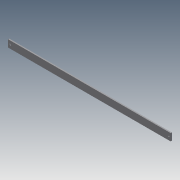
# Autodesk Inventor part: large
Saved by Autodesk Inventor 2011 (Build 150239000, 239)
## iProperties
Created: 2011-12-18
Part Number: large
Document SubType Name: Modeling
Designer: Matthew
Density: 1 g/cm^3
Author: Matthew
Autodesk Inventor part; units mm, degrees
ref_plane "YZ Plane" through (0, 0, 0) normal (1, 0, 0) x (0, 1, 0)
ref_plane "XZ Plane" through (0, 0, 0) normal (0, 1, 0) x (-1, 0, 0)
ref_plane "XY Plane" through (0, 0, 0) normal (0, 0, 1) x (1, 0, 0)
sketch "Sketch1" plane through (0, 0, 0) normal (0, 0, 1) x (1, 0, 0)
  line L0 (-31.9376, 1.7652) -> (399.8624, 1.7652)
  line L1 (399.8624, 1.7652) -> (399.8624, -10.9348)
  line L2 (399.8624, -10.9348) -> (-31.9376, -10.9348)
  line L3 (-31.9376, -10.9348) -> (-31.9376, 1.7652)
  line L4 (183.9624, -4.5848) -> (-26.4766, -4.5848)
  line L5 (-26.4766, -4.5848) -> (394.4014, -4.5848)
  circle A0 centre (-26.4766, -4.5848) radius 1.9812
  circle A1 centre (394.4014, -4.5848) radius 1.9812
  point P0 (0, 0)
  dimension "d0" = 431.8
  dimension "d1" = 12.7
  dimension "d2" = 210.439
  dimension "d3" = 420.878
  dimension "d4" = 3.9624
  dimension "d5" = 3.9624
  constraints: 12 end point, 3 parallel, 2 centre point, 2 coincident, 2 perpendicular, 1 horizontal
  measures "d0" distance of L1.end L2.end
  measures "d1" distance of L0.end L1.end
  measures "d2" distance of L4.start L4.end
  measures "d3" distance of L4.end L5.end
  measures "d4" diameter of A0
  measures "d5" diameter of A1
extrude "Extrusion1" add sketch "Sketch1" along normal blind 3.175
sketch "Sketch2" plane through (-31.9376, 1.7652, 0) normal (0, 1, 0) x (1, 0, 0)
  line L0 (0, -3.175) -> (431.8, -3.175) projected
  line L1 (431.8, 0) -> (431.8, -3.175) projected
  line L2 (0, 0) -> (431.8, 0) projected
  line L3 (0, 0) -> (0, -3.175) projected
  point P0 (31.9376, 0)
extrude "Extrusion2" add sketch "Sketch2" along normal blind 3.175
sketch "Sketch3" plane through (-31.9376, -10.9348, 0) normal (0, -1, 0) x (1, 0, 0)
  line L0 (431.8, 3.175) -> (0, 3.175) projected
  line L1 (0, 0) -> (0, 3.175) projected
  line L2 (431.8, 0) -> (0, 0) projected
  line L3 (431.8, 0) -> (431.8, 3.175) projected
  point P0 (31.9376, 0)
extrude "Extrusion3" add sketch "Sketch3" along normal blind 3.175
body "Solid1"
